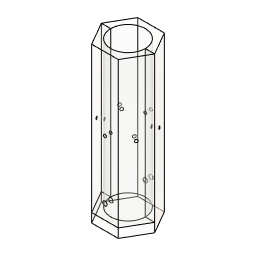
TwoPartTubeJig (Autodesk Fusion 360 design; units mm, degrees)
Autodesk Fusion 360 part; units mm, degrees
sketch "Sketch1" plane through (0, 0, 0) normal (0, 0, 1) x (1, 0, 0)
  circle A0 centre (0, 0) radius 9.525
  line L0 (-14.6647, 0) -> (-7.3323, -12.7)
  line L1 (-7.3323, -12.7) -> (7.3323, -12.7)
  line L2 (7.3323, -12.7) -> (14.6647, 0)
  line L3 (14.6647, 0) -> (7.3323, 12.7)
  line L4 (7.3323, 12.7) -> (-7.3323, 12.7)
  line L5 (-7.3323, 12.7) -> (-14.6647, 0)
  line L6 (-14.6647, 0) -> (-9.525, 0)
  line L7 (9.525, 0) -> (14.6647, 0)
  dimension "d1" = 19.05
  dimension "d2" = 25.4
  constraint coincident A0.centre origin
  constraint horizontal L4
  constraint coincident A0 L6.end
  constraint horizontal L6
  constraint coincident A0 L7.start
  constraint parallel L6 L7
  measures "d1" diameter of A0
  measures "d2" distance of L1 L4
extrude "Extrude1" add sketch "Sketch1" along normal blind 80.35 contours A0 L3 L4 L5 L6 L7 makes body 1
extrude "Extrude1'" add sketch "Sketch1" along normal blind 80.35 separate body contours A0 L0 L1 L2 L6 L7 makes body 2 in component "Component"
extrude "Extrude2" add sketch "Sketch1" against normal blind 5 bodies 1
sketch "Sketch2" plane through (0, -12.7, 0) normal (0, -1, 0) x (1, 0, 0)
  line L0 (-7.3323, 0) -> (7.3323, 0)
  line L1 (7.3323, 0) -> (7.3323, 80.35)
  line L2 (7.3323, 80.35) -> (-7.3323, 80.35)
  line L3 (-7.3323, 80.35) -> (-7.3323, 0)
  point P0 (0, 8)
  dimension "d9" = 8
  measures "d9" distance of origin P0
hole "Hole1" at (0, -12.7, 8) direction (0, 1, 0) diameter 2.3813 end through all bodies 1
hole "Hole1'" at (0, -12.7, 8) direction (0, 1, 0) diameter 2.3813 end through all bodies 1 2 in component "Component"
sketch "Sketch3" plane through (0, -12.7, 0) normal (0, -1, 0) x (1, 0, 0)
  circle A0 centre (0, 8) radius 1.1906
  line L0 (-7.3323, 0) -> (7.3323, 0)
  line L1 (7.3323, 0) -> (7.3323, 80.35)
  line L2 (7.3323, 80.35) -> (-7.3323, 80.35)
  line L3 (-7.3323, 80.35) -> (-7.3323, 0)
  line L4 (-7.3323, 0) -> (7.3323, 0)
  point P0 (0, 40.175)
  dimension "d16" = 40.175
  measures "d16" distance of P0 L4
hole "Hole2" at (0, -12.7, 40.175) direction (0, 1, 0) diameter 1.5875 end through all bodies 1
hole "Hole2'" at (0, -12.7, 40.175) direction (0, 1, 0) diameter 1.5875 end through all bodies 1 2 in component "Component"
pattern_circular "C-Pattern1" count 3 over 360 about axis through (0, 0, 1.75) along (0, 0, 1) of "Hole2"
pattern_circular "C-Pattern1'" count 3 over 360 about axis through (0, 0, 1.75) along (0, 0, 1) of "Hole2'" in component "Component"
component "Component" placed x (1, 0, 0) y (0, 1, 0) z (0, 0, 1) at (0, 0, 0)
equation "d3 = 74 mm + 0.25 in"
equation "d5 = 74 mm + 0.25 in"
equation "d11 = 3 in / 32"
equation "d14 = 3 in / 32"
equation "d16 = 37 mm + 0.125 in"
equation "d18 = 1 in / 16"
equation "d21 = 1 in / 16"
